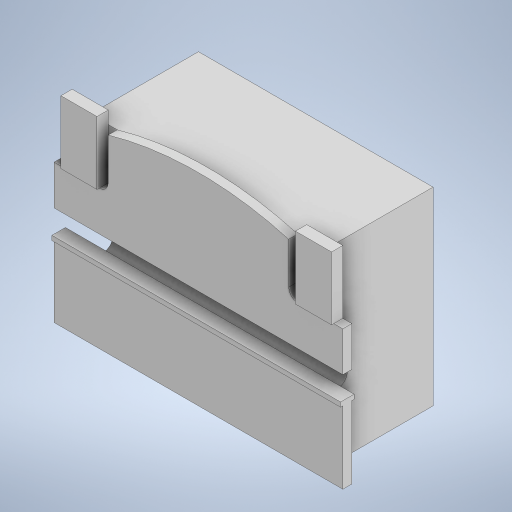
# Autodesk Inventor part: Hydraulic Sheet Metal Bending Machine PBH-135T3200 3000
Saved by Autodesk Inventor 2023.1 (Build 271208000, 208)
## iProperties
Created: 2023-08-14
Part Number: Hydraulic Sheet Metal Bending Machine PBH-135T3200 3000
Material: Generic
Document SubType Name: Modeling
Designer: admin
Density: 1 g/cm^3
Appearance: Default
Stock Number: Hydraulic Sheet Metal Bending Machine PBH-135T3200 3000
Author: admin
Autodesk Inventor part; units mm, degrees
ref_plane "YZ Plane" through (0, 0, 0) normal (1, 0, 0) x (0, 1, 0)
ref_plane "XZ Plane" through (0, 0, 0) normal (0, 1, 0) x (-1, 0, 0)
ref_plane "XY Plane" through (0, 0, 0) normal (0, 0, 1) x (1, 0, 0)
sketch "Sketch1" plane through (0, 0, 0) normal (0, 1, 0) x (-1, 0, 0)
  line L0 (1300, 0) -> (-1300, 0)
  line L1 (-1300, 0) -> (-1300, 1200)
  line L2 (-1300, 1200) -> (1300, 1200)
  line L3 (1300, 1200) -> (1300, 0)
  line L4 (1300, 0) -> (-1300, 1200) construction
  line L5 (-1300, 0) -> (1300, 1200) construction
  point P0 (0, 0)
  point P1 (0, 600)
  point P2 (0, 0)
  dimension "d0" = 2600
  dimension "d19" = 1200
  constraints: 12 end point, 3 midpoint, 2 parallel, 1 coincident, 1 horizontal, 1 perpendicular, 1 vertical alignment
  measures "d0" distance of L1.end L2.end
  measures "d19" distance of L0.end L1.end
extrude "Extrusion1" add sketch "Sketch1" along normal blind 2100
sketch "Sketch5" plane through (0, 0, 0) normal (0, 1, 0) x (-1, 0, 0)
  line L0 (-1600, 1200) -> (1600, 1200)
  line L1 (1600, 1200) -> (1600, 1300)
  line L2 (1600, 1300) -> (-1600, 1300)
  line L3 (-1600, 1300) -> (-1600, 1200)
  line L4 (-1600, 1200) -> (1600, 1300) construction
  line L5 (1600, 1200) -> (-1600, 1300) construction
  line L6 (1300, 1200) -> (-1300, 1200) projected
  point P0 (0, 0)
  point P1 (0, 1250)
  point P2 (0, 1200)
  dimension "d20" = 100
  dimension "d21" = 3200
  constraints: 12 end point, 4 midpoint, 2 parallel, 1 horizontal, 1 perpendicular
  measures "d20" distance of L2.end L0.start
  measures "d21" distance of L1.end L2.end
extrude "Extrusion5" add sketch "Sketch5" along normal blind 2240
sketch "Sketch6" plane through (-1600, 0, 1300) normal (0, 0, 1) x (1, 0, 0)
  line L0 (2900, 0) -> (300, 0) projected
  line L1 (300, 0) -> (300, 2100) projected
  line L2 (2900, 2100) -> (300, 2100) projected
  line L3 (2900, 0) -> (2900, 2100) projected
  line L4 (0, 0) -> (0, 2240) projected
  line L5 (0, 1540) -> (300, 1540)
  line L6 (300, 0) -> (300, 2100) projected
  line L7 (300, 1540) -> (500, 1540)
  arc A0 (500, 1540) -> (600, 1640) centre (500, 1640) ccw
  line L8 (600, 1640) -> (600, 2100)
  line L9 (300, 2100) -> (2900, 2100) projected
  line L10 (1600, 2100) -> (1600, -35.8904) construction
  line L11 (3200, 1540) -> (2900, 1540)
  line L12 (2900, 1540) -> (2700, 1540)
  arc A1 (2600, 1640) -> (2700, 1540) centre (2700, 1640) ccw
  line L13 (2600, 1640) -> (2600, 2100)
  line L14 (0, 2240) -> (3200, 2240) projected
  arc A2 (2600, 2100) -> (600, 2100) centre (1600, -1401.4286) ccw
  line L15 (2900, 0) -> (2900, 2100) projected
  line L16 (3200, 0) -> (3200, 2240) projected
  line L17 (3200, 0) -> (3200, 2240) projected
  point P0 (1600, 0)
  point P1 (1600, 2240)
  dimension "d24" = 700
  dimension "d25" = 600
  dimension "d26" = 100
  constraints: 14 end point, 6 point on circle, 6 symmetric about line, 5 point on line, 3 centre point, 3 tangent, 2 perpendicular, 1 midpoint, 1 vertical, 1 other
  measures "d24" distance between parallel lines of L5 L14
  measures "d25" distance between parallel lines of L4 L8
  measures "d26" radius of A0
extrude "Extrusion6" cut sketch "Sketch6" against normal up to surface (100 mm away) contours L12 A1 L13 L2 L3 | L3 L2 A2 L14 L16 L11 | L5 L4 L14 A2 L2 L1 | L1 L2 L8 A0 L7
sketch "Sketch7" plane through (0, 0, 0) normal (1, 0, 0) x (0, 1, 0)
  line L0 (0, 1300) -> (1540, 1300) projected
  line L1 (0, 0) -> (0, 1200) projected
  line L2 (2100, 0) -> (2100, 1200) projected
  line L3 (0, 1200) -> (1540, 1200) projected
  line L4 (800, 1300) -> (800, 1200)
  line L5 (0, 1200) -> (1540, 1200) projected
  line L6 (700, 1200) -> (700, 1050)
  arc A0 (700, 1050) -> (800, 950) centre (800, 1050) ccw
  line L7 (800, 950) -> (1000, 950)
  arc A1 (1000, 950) -> (1100, 1050) centre (1000, 1050) ccw
  line L8 (1100, 1050) -> (1100, 1300)
  dimension "d30" = 100
  dimension "d31" = 350
  dimension "d32" = 100
  dimension "d33" = 800
  dimension "d34" = 400
  constraints: 8 end point, 4 point on circle, 4 point on line, 4 tangent, 3 perpendicular, 2 centre point, 1 equal radius, 1 horizontal
  measures "d30" radius of A1
  measures "d31" distance between parallel lines of L0 L7
  measures "d32" distance between parallel lines of L6 L4
  measures "d33" distance between parallel lines of L1 L4
  measures "d34" distance between parallel lines of L6 L8
extrude "Extrusion7" cut sketch "Sketch7" along normal through all both and the other way through all
sketch "Sketch8" plane through (0, 0, 0) normal (1, 0, 0) x (0, 1, 0)
  line L0 (800, 1300) -> (800, 1200) projected
  line L1 (0, 1200) -> (800, 1200) projected
  line L2 (0, 1200) -> (0, 1300) projected
  line L3 (0, 1300) -> (800, 1300) projected
  line L4 (850, 1175) -> (800, 1175)
  line L5 (800, 1175) -> (800, 1325)
  line L6 (800, 1325) -> (850, 1325)
  line L7 (850, 1325) -> (850, 1175)
  line L8 (850, 1175) -> (800, 1325) construction
  line L9 (800, 1175) -> (850, 1325) construction
  line L10 (800, 1300) -> (800, 1200) projected
  point P0 (0, 0)
  point P1 (825, 1250)
  point P2 (800, 1250)
  dimension "d37" = 150
  dimension "d38" = 50
  constraints: 12 end point, 4 midpoint, 2 parallel, 1 horizontal, 1 perpendicular
  measures "d37" distance of L6.end L4.start
  measures "d38" distance of L5.end L6.end
extrude "Extrusion8" add sketch "Sketch8" along normal mid plane 3200 contours L5 L6 L7 L4 L0
sketch "Sketch9" plane through (-1300, 2100, 1200) normal (0, 0, 1) x (1, 0, 0)
  line L0 (0, -560) -> (0, 0) projected
  line L1 (0, -560) -> (200, -560) projected
  arc A0 (200, -560) -> (300, -460) centre (200, -460) ccw projected
  line L2 (300, -460) -> (300, 0) projected
  line L3 (0, 0) -> (300, 0) projected
  line L4 (2600, -560) -> (2600, 0) projected
  line L5 (2300, 0) -> (2600, 0) projected
  line L6 (2300, 0) -> (2300, -460) projected
  arc A1 (2300, -460) -> (2400, -560) centre (2400, -460) ccw projected
  line L7 (2400, -560) -> (2600, -560) projected
  line L8 (0, -560) -> (200, -560) projected
  line L9 (-200, 140) -> (200, 140)
  line L10 (200, 140) -> (200, -560)
  line L11 (200, -560) -> (-200, -560)
  line L12 (-200, -560) -> (-200, 140)
  line L13 (0, -2100) -> (0, 0) projected
  line L14 (-200, 140) -> (200, -560) construction
  line L15 (200, 140) -> (-200, -560) construction
  line L16 (2400, 140) -> (2800, 140)
  line L17 (2800, 140) -> (2800, -560)
  line L18 (2800, -560) -> (2400, -560)
  line L19 (2400, -560) -> (2400, 140)
  line L20 (2600, -560) -> (2600, 0) projected
  line L21 (2400, 140) -> (2800, -560) construction
  line L22 (2800, 140) -> (2400, -560) construction
  line L23 (-300, -2100) -> (2900, -2100) projected
  point P0 (1300, -2100)
  point P1 (0, -210)
  point P2 (2600, -210)
  point P3 (200, -560)
  dimension "d41" = 400
  dimension "d42" = 2240
  constraints: 24 end point, 4 midpoint, 4 parallel, 4 point on line, 2 collinear, 2 horizontal, 2 perpendicular
  measures "d41" distance of L16.start L16.end
  measures "d42" distance between parallel lines of L23 L16
extrude "Extrusion9" add sketch "Sketch9" along normal up to surface (125 mm away) contours L11 L12 L9 L10 L3 L0 | L0 L3 L10 L1 | L7 L19 L5 L4 | L4 L5 L19 L16 L17 L18
equation "\"d39\" = d21"
equation "\"d43\" = d21"
body "Solid1"
